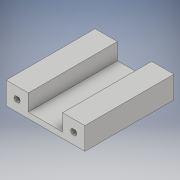
# Autodesk Inventor part: 3710-photoresistors
Saved by Autodesk Inventor 2019 (Build 230136000, 136)
## iProperties
Created: 2022-12-05
Part Number: 3710-photoresistors
Material: Generic
Document SubType Name: Modeling
Designer: Ella Moss
Density: 1 g/cm^3
Appearance: Default
Author: Ella Moss
Autodesk Inventor part; units mm, degrees
ref_plane "YZ Plane" through (0, 0, 0) normal (1, 0, 0) x (0, 1, 0)
ref_plane "XZ Plane" through (0, 0, 0) normal (0, 1, 0) x (-1, 0, 0)
ref_plane "XY Plane" through (0, 0, 0) normal (0, 0, 1) x (1, 0, 0)
sketch "Sketch1" plane through (0, 0, 0) normal (0, 0, 1) x (1, 0, 0)
  point P0 (0, 0)
sketch "Sketch2" plane through (0, 0, 0) normal (0, 0, 1) x (1, 0, 0)
  line L0 (-35.4076, 20) -> (35.4076, 20)
  line L1 (35.4076, 20) -> (35.4076, 0)
  line L2 (35.4076, 0) -> (-35.4076, 0)
  line L3 (-35.4076, 0) -> (-35.4076, 20)
  line L4 (0, 0) -> (0, 20)
  line L5 (24.0038, 12.27) -> (26.7962, 12.27)
  line L6 (24.0038, 7.73) -> (26.7962, 7.73)
  arc A0 (26.7962, 7.73) -> (26.7962, 12.27) centre (25.4, 10) ccw
  arc A1 (24.0038, 12.27) -> (24.0038, 7.73) centre (25.4, 10) ccw
  line L7 (-26.7962, 12.27) -> (-24.0038, 12.27)
  line L8 (-26.7962, 7.73) -> (-24.0038, 7.73)
  arc A2 (-24.0038, 7.73) -> (-24.0038, 12.27) centre (-25.4, 10) ccw
  arc A3 (-26.7962, 12.27) -> (-26.7962, 7.73) centre (-25.4, 10) ccw
  line L9 (-15.4, 20) -> (-15.4, 5.08)
  line L10 (-15.4, 5.08) -> (15.4, 5.08)
  line L11 (15.4, 5.08) -> (15.4, 20)
  dimension "d0" = 20
  dimension "d5" = 10.0076
  dimension "d9" = 4.54
  dimension "d10" = 116.812
  dimension "d11" = 116.812
  dimension "d12" = 4.54
  dimension "d13" = 116.812
  dimension "d14" = 116.812
  dimension "d15" = 10
  dimension "d16" = 50.8
  dimension "d17" = 5.08
  dimension "d18" = 10
  constraints: 24 end point, 8 point on circle, 6 parallel, 4 centre point, 3 horizontal, 3 perpendicular, 2 midpoint, 2 point on line, 1 coincident, 1 horizontal alignment, 1 symmetric about line, 1 vertical, 1 other
  measures "d0" distance between parallel lines of L2 L0
  measures "d5" distance from line of L1 A0.centre
  measures "d9" distance between parallel lines of L5 L6
  measures "d12" distance between parallel lines of L7 L8
  measures "d15" distance from line of L2 A2.centre
  measures "d16" distance of A0.centre A2.centre
  measures "d17" distance between parallel lines of L2 L10
  measures "d18" distance from line of A0.centre L11
extrude "Extrusion1" add sketch "Sketch2" along normal blind 80 contours L0 L9 L10 L4 L2 L3 | L4 L10 L11 L0 L1 L2
body "Solid1"
